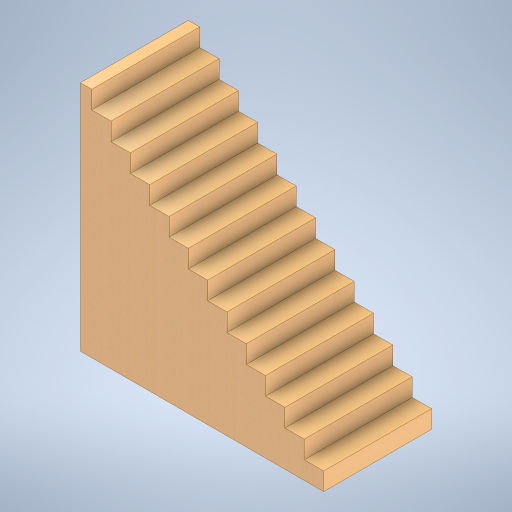
# Autodesk Inventor part: Stairs_Between_Basement_And_First_Floor
Saved by Autodesk Inventor 2024 (Build 280153000, 153)
## iProperties
Created: 2023-05-16
Part Number: Stairs_Between_Basement_And_First_Floor
Material: Wood (Oak)
Document SubType Name: Modeling
Designer: Tom
Density: 0.76 g/cm^3
Appearance: Yellow Pine - Solid Stained Light Low Gloss
Author: Tom
Autodesk Inventor part; units mm, degrees
ref_plane "YZ Plane" through (0, 0, 0) normal (1, 0, 0) x (0, 1, 0)
ref_plane "XZ Plane" through (0, 0, 0) normal (0, 1, 0) x (-1, 0, 0)
ref_plane "XY Plane" through (0, 0, 0) normal (0, 0, 1) x (1, 0, 0)
sketch "Sketch1" plane through (0, 0, 0) normal (0, 0, 1) x (1, 0, 0)
  line L0 (-184.15, 170.4731) -> (-184.15, 340.9462)
  line L1 (-184.15, 340.9462) -> (-368.3, 340.9462)
  line L2 (-368.3, 340.9462) -> (-368.3, 511.4192)
  line L3 (-368.3, 511.4192) -> (-552.45, 511.4192)
  line L4 (-552.45, 511.4192) -> (-552.45, 681.8923)
  line L5 (-552.45, 681.8923) -> (-736.6, 681.8923)
  line L6 (-736.6, 681.8923) -> (-736.6, 852.3654)
  line L7 (-736.6, 852.3654) -> (-920.75, 852.3654)
  line L8 (-920.75, 852.3654) -> (-920.75, 1022.8385)
  line L9 (-920.75, 1022.8385) -> (-1104.9, 1022.8385)
  line L10 (-1104.9, 1022.8385) -> (-1104.9, 1193.3115)
  line L11 (-1104.9, 1193.3115) -> (-1289.05, 1193.3115)
  line L12 (-1289.05, 1193.3115) -> (-1289.05, 1363.7846)
  line L13 (-1289.05, 1363.7846) -> (-1473.2, 1363.7846)
  line L14 (-1473.2, 1363.7846) -> (-1473.2, 1534.2577)
  line L15 (-1473.2, 1534.2577) -> (-1657.35, 1534.2577)
  line L16 (-1657.35, 1534.2577) -> (-1657.35, 1704.7308)
  line L17 (-1657.35, 1704.7308) -> (-1841.5, 1704.7308)
  line L18 (-1841.5, 1704.7308) -> (-1841.5, 1875.2038)
  line L19 (-1841.5, 1875.2038) -> (-2025.65, 1875.2038)
  line L20 (-2025.65, 1875.2038) -> (-2025.65, 2045.6769)
  line L21 (-2025.65, 2045.6769) -> (-2209.8, 2045.6769)
  line L22 (-2209.8, 2045.6769) -> (-2209.8, 2216.15)
  line L23 (-2209.8, 2216.15) -> (-2317.75, 2216.15)
  line L24 (-2317.75, 2216.15) -> (-2317.75, 0)
  line L25 (-184.15, 170.4731) -> (0, 170.4731)
  line L26 (0, 170.4731) -> (0, 0)
  line L27 (0, 0) -> (-2317.75, 0)
  point P0 (-2590.1533, 586.4349)
  dimension "d3" = 107.95
  dimension "d9" = 2216.15
  dimension "d10" = 2317.75
  constraints: 56 end point, 24 perpendicular, 23 parallel, 3 horizontal, 1 coincident, 1 vertical
  measures "d3" distance between parallel lines of L24 L22
  measures "d9" distance of L23.end L24.end
  measures "d10" distance of L26.end L24.end
extrude "Extrusion1" add sketch "Sketch1" along normal blind 1028.7
body "Solid1"
